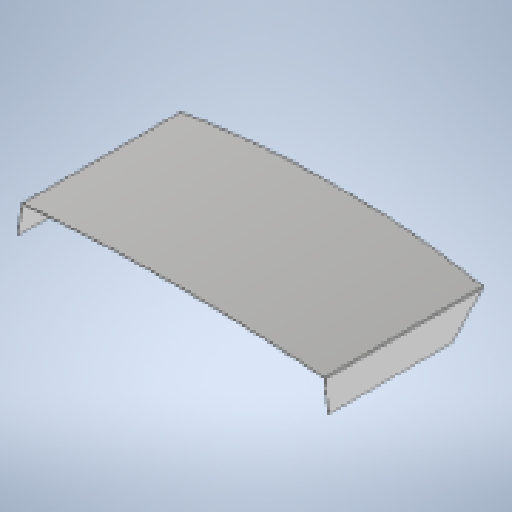
# Autodesk Inventor part: МОО 012 лист спина 2
Saved by Autodesk Inventor 2024.2 (Build 282272000, 272)
## iProperties
Created: 2024-04-18
Part Number: МОО 012 лист спина 2
Material: Stainless Steel AISI 304
Document SubType Name: Sheet Metal
Designer: admin
Stock Number: МОО 010 лист спина 1
Mass: 48037.2 g
Surface Area: 40211.1 cm^2
Volume: 6004.65 cm^3
Density: 8 g/cm^3
Flat Pattern Width: 178.583 cm
Flat Pattern Length: 81.8 cm
Flat Pattern Area: 14608.1 cm^2
Sheet Metal Rule: Default_mm
Sheet Metal Width: 1785,833 mm
Sheet Metal Length: 818,000 mm
Sheet Metal Area: 1460811,371 mm^2
Appearance: Default
Поясница_радиус: 8688,266 mm
Author: admin
Autodesk Inventor part; units mm, degrees
ref_plane "YZ Plane" through (0, 0, 0) normal (1, 0, 0) x (0, 1, 0)
ref_plane "XZ Plane" through (0, 0, 0) normal (0, 1, 0) x (-1, 0, 0)
ref_plane "XY Plane" through (0, 0, 0) normal (0, 0, 1) x (1, 0, 0)
sketch "Sketch1" plane through (0, 0, 0) normal (0, 0, 1) x (1, 0, 0)
  line L0 (-785, -32) -> (785, -32) construction
  line L1 (785, -32) -> (785, 0) construction
  line L2 (785, 0) -> (-785, 0) construction
  line L3 (-785, 0) -> (-785, -32) construction
  arc A0 (745, -32) -> (-745, -32) centre (0, -8688.2656) ccw
  arc A1 (-745, -32) -> (-747.7204, -34.6233) centre (-744.7428, -34.989) ccw
  line L4 (-747.7204, -34.6233) -> (-764.904, -174.5723)
  arc A2 (747.7204, -34.6233) -> (745, -32) centre (744.7428, -34.989) ccw
  line L5 (747.7204, -34.6233) -> (764.904, -174.5723)
  line L6 (0, 0) -> (0, -32) construction
  dimension "d0" = 1570
  dimension "d1" = 32
  dimension "d2" = 40
  dimension "d14" = 3
  dimension "d15" = 141
  dimension "d16" = 97
  dimension "d21" = 8688.2656
  measures "d0" distance of L2.end L1.end
  measures "d1" distance of L1.end L0.end
  measures "d2" distance of L0.start A0.end
  measures "d14" radius of A1
  measures "d15" distance of L4.start L4.end
  measures "d16" angle of L4 L0
  measures "d21" radius of A0
contour flange "Contour Flange1" sketch "Sketch1" thickness 3 bend radius 3 width 818 along (0, 0, 1) mid plane no both sides no wall seen from (756.3122, -104.5978, 0) lies toward (0.9925462, 0.1218693, 0) curves L5 A2 A0 A1 L4
bend "Bend1"
corner "Corner1"
sketch "Sketch2" plane through (0, 0, 0) normal (1, 0, 0) x (0, 1, 0)
  line L0 (3, 0) -> (3, 818) construction
  line L1 (0, 818) -> (-174.5723, 609.9528)
  line L2 (3, 0) -> (-29.011, 0) projected
  line L3 (0, 0) -> (-174.5723, 208.0472)
  line L4 (-174.5723, 0) -> (-174.5723, 818) projected
  line L5 (3, 818) -> (-174.5723, 818)
  line L6 (-174.5723, 0) -> (3, 0)
  line L7 (0, 0) -> (-32, 0) projected
  line L8 (-32, 818) -> (0, 818) projected
  line L9 (0, 0) -> (0, 818) construction
  point P0 (-29.011, 0)
  point P1 (0, 0)
  dimension "d20" = 40
  constraints: 10 end point, 2 perpendicular, 2 point on line, 1 equal length
  measures "d20" angle of L4 L3
extrude "Extrusion1" cut sketch "Sketch2" along normal through all both and the other way through all contours L2 L6 L4 L3
equation "\"d14\" = BendRadius"
equation "\"d3\" = Thickness"
equation "\"d4\" = BendReliefWidth"
equation "\"d5\" = BendReliefDepth"
equation "\"d6\" = MinimumRemnant"
equation "\"d7\" = TransitionRadius"
equation "\"d9\" = BendRadius"
equation "\"d11\" = CornerReliefSize"
equation "\"d12\" = GapSize"
equation "\"d13\" = JacobiRadiusSize"
equation "\"BendRadius\" = Thickness"
equation "\"BendReliefWidth\" = Thickness"
equation "\"BendReliefDepth\" = 0.5 * Thickness"
equation "\"CornerReliefSize\" = 4 * Thickness"
equation "\"MinimumRemnant\" = 2 * Thickness"
equation "\"TransitionRadius\" = BendRadius"
equation "\"JacobiRadiusSize\" = BendRadius"
equation "\"GapSize\" = Thickness"
equation "\"Поясница_радиус\" = d21"
equation "\"Thickness\" = 3"
body "Solid1"
